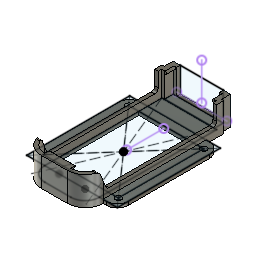
E8372 Holder (Autodesk Fusion 360 design; units mm, degrees)
Autodesk Fusion 360 part; units mm, degrees
note: some values were not read from the file. Chosen so that the rebuilt part matches the saved one: which face or edge a step refers to; which pieces of a blend or face edit are solid.
sketch "Base" plane through (0, 0, 0) normal (0, 0, 1) x (1, 0, 0)
  line L0 (15.3, 36.75) -> (-15.3, 36.75)
  line L1 (-15.3, 36.75) -> (-15.3, -28.75)
  line L2 (-7.3, -36.75) -> (7.3, -36.75)
  line L3 (15.3, -28.75) -> (15.3, 36.75)
  line L4 (15.3, 36.75) -> (-15.3, -36.75) construction
  line L5 (-15.3, 36.75) -> (15.3, -36.75) construction
  arc A0 (-15.3, -28.75) -> (-7.3, -36.75) centre (-7.3, -28.75) ccw
  arc A1 (7.3, -36.75) -> (15.3, -28.75) centre (7.3, -28.75) ccw
  line L6 (-14, 36.75) -> (14, 36.75)
  line L7 (14, 36.75) -> (14, 41.75)
  line L8 (14, 41.75) -> (-14, 41.75)
  line L9 (-14, 41.75) -> (-14, 36.75)
  line L10 (0, 1.75) -> (0, 22.5)
  line L11 (25.3, -28.75) -> (-25.3, -28.75)
  line L12 (-25.3, -28.75) -> (-25.3, 28.75)
  line L13 (-25.3, 28.75) -> (25.3, 28.75)
  line L14 (25.3, 28.75) -> (25.3, -28.75)
  line L15 (25.3, -28.75) -> (-25.3, 28.75) construction
  line L16 (-25.3, -28.75) -> (25.3, 28.75) construction
  line L17 (21, 23.8636) -> (-21, 23.8636)
  line L18 (-21, 23.8636) -> (-21, -23.8636)
  line L19 (-21, -23.8636) -> (21, -23.8636)
  line L20 (21, -23.8636) -> (21, 23.8636)
  line L21 (21, 23.8636) -> (-21, -23.8636) construction
  line L22 (-21, 23.8636) -> (21, -23.8636) construction
  dimension "d1" = 30.6
  dimension "d2" = 73.5
  dimension "d3" = 8
  dimension "d4" = 28
  dimension "d5" = 5
  dimension "d12" = 10
  dimension "d13" = 42
  constraint horizontal L0
  constraint perpendicular L0 L1
  constraint parallel L0 L2
  constraint parallel L1 L3
  constraint coincident L4 origin
  constraint coincident L5 origin
  constraint coincident L4.end L1
  constraint coincident L4.end L2
  constraint tangent L1 A0
  constraint tangent L2 A0
  constraint coincident L5.end L2
  constraint coincident L5.end L3
  constraint tangent L2 A1
  constraint tangent L3 A1
  constraint equal A0 A1
  constraint horizontal L6
  constraint vertical L7
  constraint horizontal L8
  constraint vertical L9
  constraint symmetric L7 L9 L10
  constraint collinear L0 L6
  constraint horizontal L11
  constraint perpendicular L11 L12
  constraint parallel L11 L13
  constraint parallel L12 L14
  constraint coincident L15 origin
  constraint coincident L16 origin
  constraint coincident A1.centre L11
  constraint horizontal L17
  constraint perpendicular L17 L18
  constraint parallel L17 L19
  constraint parallel L18 L20
  constraint coincident L16 L17.start
  constraint coincident L21 origin
  constraint coincident L22 origin
  measures "d1" distance of L4.end L5.end
  measures "d2" distance of L0.end L4.end
  measures "d3" radius of A0
  measures "d4" distance of L6.start L6.end
  measures "d5" distance of L6.start L8.end
  measures "d12" distance of L1 L12
  measures "d13" distance of L18.end L19.end
extrude "Extrude1" add sketch "Base" along normal blind 14 contours L0 L1 L3 L6 L13 | L0 L6 L7 L8 L9 | L1 L3 L13 L17 | L1 L3 L17 L19 | L1 L3 L11 L19 | L2 A0 A1 L11
shell "Shell1" thickness 2 outward yes removed faces 1 at (4.6667, -6.9167, 14)
sketch "end" plane through (0, 43.75, 0) normal (0, 1, 0) x (-1, 0, 0)
  line L0 (-16, -2) -> (16, -2)
  line L1 (16, -2) -> (16, 14)
  line L2 (16, 14) -> (-16, 14)
  line L3 (-16, 14) -> (-16, -2)
  line L4 (-12, 0) -> (12, 0)
  line L5 (12, 0) -> (12, 14)
  line L6 (12, 14) -> (-12, 14)
  line L7 (-12, 14) -> (-12, 0)
  line L8 (-14, 0) -> (14, 0)
  line L9 (0, 1.75) -> (0, 22.5)
  dimension "d9" = 24
  constraint horizontal L4
  constraint vertical L5
  constraint horizontal L6
  constraint vertical L7
  constraint collinear L4 L8
  constraint symmetric L5 L7 L9
  constraint collinear L2 L6
  measures "d9" distance of L5 L7
extrude "Extrude2" cut sketch "end" against normal blind 2 contours L2 L4 L5 L6 L7 L8
extrude "Extrude3" add sketch "Base" against normal blind 2 contours L3 L11 L13 L14 L17 L19 L20 | L3 L17 L19 L20 | L1 L11 L12 L13 L17 L18 L19 | L1 L17 L18 L19
extrude "Extrude4" cut sketch "Base" against normal blind 2 contours L1 L3 L17 L19
hole "Hole1" at (-21, 23.8636, 0) at (21, 23.8636, 0) at (21, -23.8636, 0) at (-21, -23.8636, 0) direction (0, 0, -1) diameter 3.5 depth 2 tip angle 180
sketch "Side" plane through (-17.3, 0, 0) normal (-1, 0, 0) x (0, -1, 0)
  line L0 (-28.75, 0) -> (28.75, 0)
  line L1 (28.75, 0) -> (28.75, 14)
  line L2 (28.75, 14) -> (-38.75, 14)
  line L3 (-38.75, 14) -> (-38.75, -2)
  line L4 (-38.75, -2) -> (-28.75, -2)
  line L5 (-28.75, -2) -> (-28.75, 0)
  line L6 (-34.75, 14) -> (26.75, 14)
  line L7 (26.75, 14) -> (26.75, 4)
  line L8 (26.75, 4) -> (-34.75, 4)
  line L9 (-34.75, 4) -> (-34.75, 14)
  line L10 (28.75, 0) -> (-28.75, 0)
  dimension "d21" = 2
  dimension "d22" = 4
  dimension "d23" = 4
  constraint horizontal L6
  constraint vertical L7
  constraint horizontal L8
  constraint vertical L9
  constraint coincident L2 L6.start
  measures "d21" distance of L1 L7
  measures "d22" distance of L3 L9
  measures "d23" distance of L8 L10
extrude "Extrude5" cut sketch "Side" against normal through all contours L2 L6 L7 L8 L9
sketch "Lip" plane through (0, -38.75, 0) normal (0, -1, 0) x (1, 0, 0)
  line L0 (-7.3, -2) -> (7.3, -2)
  line L1 (7.3, -2) -> (7.3, 14)
  line L2 (7.3, 14) -> (-7.3, 14)
  line L3 (-7.3, 14) -> (-7.3, -2)
  line L4 (17.3, 14) -> (17.3, 4)
  line L5 (-17.3, 4) -> (-17.3, 14)
  line L6 (17.3, 12.2) -> (-17.3, 12.2)
  line L7 (-12, 14) -> (12, 14)
  dimension "d25" = 1.8
  constraint coincident L4 L6.start
  constraint coincident L5 L6.end
  constraint perpendicular L3 L6
  measures "d25" distance of L6 L7
extrude "Extrude6" add sketch "Lip" against normal blind 2.5 from surface at -2 contours L1 L2 L3 L6 L7
chamfer "Chamfer1" distance 1.5 distance2 2 1 edges at (0, -34.25, 12.2) measured on face at (-2.4333, -34.25, 13.4)
box "BoxPrimitive1" add length 2.5 width 5 height 1.5 placed x (0, 0, -1) y (0, -1, 0) z (-1, 0, 0) at (14, 41.8, 14)
chamfer "Chamfer2" distance 1.5 distance2 1.5 1 edges at (12.5, 39.275, 11.5) measured on face at (12.5, 38.45, 13.1667)
chamfer "Chamfer4" distance 1 distance2 1 1 edges at (12.5, 39.275, 14) measured on face at (12.5, 38.45, 13.6666)
mirror "Mirror1" about plane through (0, 0, 0) normal (1, 0, 0) of "BoxPrimitive1", "Chamfer2", "Chamfer4"
fillet "Fillet1" radius 6 4 edges at (-25.3, 28.75, -1) (25.3, 28.75, -1) (25.3, -28.75, -1) (-25.3, -28.75, -1)
chamfer "Chamfer5" distance 4 distance2 10 2 edges at (-16.3, -26.75, 14) (16.3, -26.75, 14) measured on face at (-2.4333, -35.0833, 14) measured on face at (-2.4333, -35.0833, 14)
fillet "Fillet2" radius 2 2 edges at (16.072, -30.75, 14) (-16.072, -30.75, 14)
fillet "Fillet3" radius 2 6 edges at (16.3, -26.75, 4.002) (16.3, -26.75, 4) (16.3, 34.75, 4) (-16.3, -26.75, 4.002) (-16.3, -26.75, 4) (-16.3, 34.75, 4)
named bodies: "E8372 mount"
